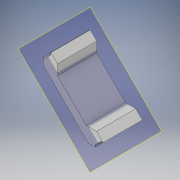
# Autodesk Inventor part: 20_Cube_Insert_Mirror_Holder_wLogo_v3
Saved by Autodesk Inventor 2019 (Build 230136000, 136)
## iProperties
Created: 2019-07-22
Part Number: 20_Cube_Insert_Mirror_Holder_wLogo_v3
Material: Generic
Document SubType Name: Modeling
Designer: diederichbenedict
Density: 1 g/cm^3
Appearance: Default
Mass: 13.6419 g
Surface Area: 50.8514 cm^2
Volume: 13.6419 cm^3
Author: diederichbenedict
Autodesk Inventor part; units mm, degrees
ref_plane "YZ Plane" through (0, 0, 0) normal (1, 0, 0) x (0, 1, 0)
ref_plane "XZ Plane" through (0, 0, 0) normal (0, 1, 0) x (-1, 0, 0)
ref_plane "XY Plane" through (0, 0, 0) normal (0, 0, 1) x (1, 0, 0)
sketch "Sketch1" plane through (0, 0, 0) normal (0, 0, 1) x (1, 0, 0)
  line L0 (-16.9, 21.4) -> (-16.9, 16.9) construction
  arc A0 (-22.9, 19.9) -> (-19.9, 22.9) centre (-19.9, 19.9) ccw construction
  line L1 (-16.9, 16.9) -> (16.9, 16.9) construction
  line L2 (16.9, 16.9) -> (16.9, -16.9) construction
  line L3 (16.9, -16.9) -> (-16.9, -16.9) construction
  line L4 (-16.9, -16.9) -> (-16.9, 16.9) construction
  arc A1 (22.9, -19.9) -> (19.9, -22.9) centre (19.9, -19.9) ccw construction
  line L5 (22.9, 19.9) -> (22.9, -19.9) construction
  arc A2 (19.9, 22.9) -> (22.9, 19.9) centre (19.9, 19.9) ccw construction
  line L6 (-19.9, 22.9) -> (19.9, 22.9) construction
  arc A3 (-22.9, 19.9) -> (-19.9, 22.9) centre (-19.9, 19.9) ccw construction
  line L7 (-22.9, -19.9) -> (-22.9, 19.9) construction
  arc A4 (-19.9, -22.9) -> (-22.9, -19.9) centre (-19.9, -19.9) ccw construction
  line L8 (19.9, -22.9) -> (-19.9, -22.9) construction
  line L9 (-21.4, 16.9) -> (-16.9, 16.9) construction
  line L10 (-16.9, -16.9) -> (-21.4, -16.9) construction
  line L11 (-16.9, -16.9) -> (-16.9, -21.4) construction
  line L12 (16.9, -21.4) -> (16.9, -16.9) construction
  line L13 (21.4, -16.9) -> (16.9, -16.9) construction
  line L14 (16.9, 16.9) -> (21.4, 16.9) construction
  line L15 (16.9, 16.9) -> (16.9, 21.4) construction
  line L16 (-16.8009, 21.2415) -> (21.2415, -16.8009)
  line L17 (21.2415, -16.8009) -> (16.8009, -21.2415)
  line L18 (16.8009, -21.2415) -> (-21.2415, 16.8009)
  line L19 (-21.2415, 16.8009) -> (-16.8009, 21.2415)
  line L20 (-16.8009, 21.2415) -> (16.8009, -21.2415) construction
  line L21 (21.2415, -16.8009) -> (-21.2415, 16.8009) construction
  line L22 (-16.8009, 21.2415) -> (36.9991, 21.2415) construction
  line L23 (-21.2415, 16.8009) -> (-22.9, 16.8009)
  line L24 (16.8009, -21.2415) -> (16.8009, -22.9)
  line L25 (16.8009, -22.9) -> (-22.9, 16.8009)
  line L26 (-16.8009, 21.2415) -> (-16.8009, 22.9)
  line L27 (21.2415, -16.8009) -> (22.9, -16.8009)
  line L28 (22.9, -16.8009) -> (-16.8009, 22.9)
  line L29 (-22.9, 16.8009) -> (-22.9, 11.5863)
  line L30 (16.8009, -22.9) -> (11.5863, -22.9)
  line L31 (-22.9, 11.5863) -> (11.5863, -22.9)
  point P0 (0, 0)
  dimension "d0" = 53.8
  dimension "d1" = 45
  dimension "d2" = 6.28
  dimension "d5" = 8
  constraints: 32 end point, 6 point on line, 4 parallel, 4 perpendicular, 2 midpoint, 1 equal length, 1 horizontal
  measures "d0" distance of L16.start L16.end
  measures "d1" angle of L16 L22
  measures "d2" distance of L16.end L17.end
  measures "d5" distance from line of L31 point (0, 0)
extrude "Extrusion1" add sketch "Sketch1" along normal blind 30
ref_plane "Work Plane1" through (16.9, -16.9, -8) normal (-0.7071068, -0.7071068, 0) x (0, 0, 1)
sketch "Sketch7" plane through (0, 0, 30) normal (0, 0, 1) x (1, 0, 0)
  line L0 (21.2415, -16.8009) -> (22.9, -16.8009) projected
  line L1 (22.9, -16.8009) -> (-16.8009, 22.9) projected
  line L2 (-16.8009, 22.9) -> (-16.8009, 21.2415) projected
  line L3 (-16.8009, 21.2415) -> (-21.2415, 16.8009) projected
  line L4 (-21.2415, 16.8009) -> (-22.9, 16.8009) projected
  line L5 (-22.9, 16.8009) -> (-22.9, 11.5863) projected
  line L6 (-22.9, 11.5863) -> (11.5863, -22.9) projected
  line L7 (11.5863, -22.9) -> (16.8009, -22.9) projected
  line L8 (16.8009, -22.9) -> (16.8009, -21.2415) projected
  line L9 (16.8009, -21.2415) -> (21.2415, -16.8009) projected
  line L10 (3.0496, 3.0496) -> (-5.6569, -5.6569)
  line L11 (-22.9, 11.5863) -> (11.5863, -22.9) projected
  line L12 (17.9785, -3.9418) -> (10.0409, -11.8794)
  line L13 (10.0409, -11.8794) -> (-11.8794, 10.0409)
  line L14 (-11.8794, 10.0409) -> (-3.9418, 17.9785)
  line L15 (-3.9418, 17.9785) -> (17.9785, -3.9418)
  line L16 (17.9785, -3.9418) -> (-11.8794, 10.0409) construction
  line L17 (10.0409, -11.8794) -> (-3.9418, 17.9785) construction
  line L18 (-11.8794, 10.0409) -> (-11.8794, 17.9785)
  line L19 (22.9, -16.8009) -> (-16.8009, 22.9) projected
  line L20 (10.0409, -11.8794) -> (17.9785, -11.8794)
  point P0 (0, 0)
  dimension "d28" = 31
  dimension "d29" = 1.3
  constraints: 18 end point, 4 midpoint, 2 parallel, 2 perpendicular, 2 point on line, 1 vertical
  measures "d28" distance of L12.end L13.end
  measures "d29" distance from line of L13 point (0, 0)
extrude "Extrusion7" cut sketch "Sketch7" against normal through all contours L20 L12 L1 | L12 L13 L10 L1 | L1 L14 L15 L12 | L10 L13 L14 L1 | L14 L18 L1
sketch "Sketch10" plane through (11.5863, -22.9, 30) normal (-0.7071068, -0.7071068, 0) x (-0.7071068, 0.7071068, 0)
  line L0 (1.6838, 16.5215) -> (7.0744, 16.5215) construction
  line L1 (7.0744, 16.5215) -> (7.0744, 10.5304) construction
  line L2 (7.0744, 10.5304) -> (1.6838, 10.5304) construction
  line L3 (1.6838, 10.5304) -> (1.6838, 6.839) construction
  line L4 (1.6838, 6.839) -> (6.7206, 6.839) construction
  line L5 (6.7206, 6.839) -> (6.7206, 1.2092) construction
  line L6 (6.7206, 1.2092) -> (1.6838, 1.2092) construction
  line L7 (1.6838, 1.2092) -> (1.6838, -3.423) construction
  line L8 (1.6838, -3.423) -> (34.6838, -3.423) construction
  line L9 (34.6838, 30.377) -> (1.6838, 30.377) construction
  line L10 (1.6838, 30.377) -> (1.6838, 26.2152) construction
  line L11 (1.6838, 26.2152) -> (7.1181, 26.2152) construction
  line L12 (7.1181, 26.2152) -> (7.1181, 20.0634) construction
  line L13 (7.1181, 20.0634) -> (1.6838, 20.0634) construction
  line L14 (1.6838, 20.0634) -> (1.6838, 16.5215) construction
  line L15 (7.0744, 13.526) -> (34.6838, 13.477) construction
  line L16 (1.6838, 30.377) -> (36.6838, 30.377) construction
  line L17 (36.6838, -3.423) -> (1.6838, -3.423) construction
  line L18 (15.7252, 20) -> (15.7252, 10)
  line L19 (15.7252, 10) -> (24.3855, 5)
  line L20 (15.7252, 20) -> (17.2252, 19.134)
  line L21 (17.2252, 19.134) -> (17.2252, 10.866)
  line L22 (17.2252, 10.866) -> (22.8855, 7.5981)
  line L23 (22.8855, 7.5981) -> (22.8855, 15.866)
  line L24 (22.8855, 15.866) -> (24.3855, 15)
  line L25 (24.3855, 15) -> (24.3855, 5)
  line L26 (34.6838, 30.377) -> (34.6838, -3.423)
  line L27 (24.3855, 31.8785) -> (24.3855, -1.9215) construction
  line L28 (1.6838, -3.423) -> (34.6838, -3.423) construction
  line L29 (34.6838, 30.377) -> (34.6838, 30.377) construction
  line L30 (34.6838, 30.377) -> (34.6838, -3.423) construction
  line L31 (34.6838, -3.423) -> (34.6838, -3.423) construction
  line L32 (34.6838, -3.423) -> (34.6838, 30.377) construction
  line L33 (48.771, 30) -> (0, 30) construction
  line L34 (0, 30) -> (0, 0) construction
  line L35 (48.771, 0) -> (0, 0) construction
  line L36 (48.771, 30) -> (48.771, 0) construction
  line L37 (24.3855, 30) -> (24.3855, 0) construction
  line L38 (48.771, 0) -> (0, 0) construction
  line L39 (48.771, 30) -> (48.771, 0) construction
  line L40 (48.771, 15) -> (0, 15) construction
  line L41 (0, 30) -> (0, 0) construction
  point P0 (24.3855, 15)
  dimension "d40" = 1.5
  dimension "d41" = 1.5
  dimension "d42" = 1.5
  dimension "d43" = 10
  dimension "d44" = 10
  constraints: 70 end point, 6 midpoint, 4 parallel, 3 collinear, 1 perpendicular, 1 vertical
  measures "d40" distance between parallel lines of L21 L18
  measures "d41" distance between parallel lines of L25 L23
  measures "d42" distance between parallel lines of L19 L22
  measures "d43" distance of L18.start L18.end
  measures "d44" distance of L18.end L19.end
emboss "Emboss1" sketch "Sketch10" operation cut depth 1 direction (0.7071068, 0.7071068, 0)
sketch "Sketch11" plane through (11.5863, -22.9, 30) normal (-0.7071068, -0.7071068, 0) x (-0.7071068, 0.7071068, 0)
  line L0 (17.2252, 10.866) -> (22.8855, 7.5981) construction
  line L1 (22.8855, 7.5981) -> (22.8855, 15.866) construction
  line L2 (22.8855, 15.866) -> (24.3855, 15) construction
  line L3 (24.3855, 15) -> (24.3855, 5) construction
  line L4 (24.3855, 5) -> (15.7252, 10) construction
  line L5 (15.7252, 10) -> (15.7252, 20) construction
  line L6 (15.7252, 20) -> (17.2252, 19.134) construction
  line L7 (17.2252, 19.134) -> (17.2252, 10.866) construction
  line L8 (48.771, 30) -> (0, 30) construction
  line L9 (0, 30) -> (0, 0) construction
  line L10 (48.771, 0) -> (0, 0) construction
  line L11 (48.771, 30) -> (48.771, 0) construction
  line L12 (15.7252, 20) -> (17.2252, 19.134) construction
  line L13 (17.2252, 19.134) -> (17.2252, 10.866) construction
  line L14 (17.2252, 10.866) -> (22.8855, 7.5981) construction
  line L15 (22.8855, 7.5981) -> (22.8855, 15.866) construction
  line L16 (22.8855, 15.866) -> (24.3855, 15) construction
  line L17 (24.3855, 15) -> (24.3855, 5) construction
  line L18 (24.3855, 5) -> (15.7252, 10) construction
  line L19 (15.7252, 10) -> (15.7252, 20) construction
  line L20 (15.5651, 18.4016) -> (15.5, -16.9) construction
  line L21 (15.5651, 18.4016) -> (-17.5, 16.9) construction
  line L22 (-17.5, 16.9) -> (-17.5, 12.7382) construction
  line L23 (-17.5, 12.7382) -> (-12.0658, 12.7382) construction
  line L24 (-12.0658, 12.7382) -> (-12.0658, 6.5864) construction
  line L25 (-12.0658, 6.5864) -> (-17.5, 6.5864) construction
  line L26 (-17.5, 6.5864) -> (-17.5, 3.0446) construction
  line L27 (-17.5, 3.0446) -> (-12.1095, 3.0446) construction
  line L28 (-12.1095, 3.0446) -> (-12.1095, -2.9465) construction
  line L29 (-12.1095, -2.9465) -> (-17.5, -2.9465) construction
  line L30 (-17.5, -2.9465) -> (-17.5, -6.638) construction
  line L31 (-17.5, -6.638) -> (-12.4632, -6.638) construction
  line L32 (-12.4632, -6.638) -> (-12.4632, -12.2678) construction
  line L33 (-12.4632, -12.2678) -> (-17.5, -12.2678) construction
  line L34 (-17.5, -12.2678) -> (-17.5, -16.9) construction
  line L35 (-17.5, -16.9) -> (15.5, -16.9) construction
  line L36 (-12.1095, 0.049) -> (15.5326, 0.7508) construction
  line L37 (15.5, -16.9) -> (15.5651, 18.4016) construction
  line L38 (1.91, 17.7815) -> (1.91, -16.9) construction
  line L39 (15.5, -16.9) -> (-17.5, -16.9) construction
  line L40 (22.8855, 7.5981) -> (22.8855, 15.866) construction
  line L41 (17.2252, 19.134) -> (17.2252, 10.866)
  line L42 (17.2252, 10.866) -> (22.8855, 7.5981)
  line L43 (17.2252, 19.134) -> (17.2252, 10.866)
  line L44 (17.2252, 10.866) -> (22.8855, 7.5981)
  line L45 (22.8855, 7.5981) -> (22.8855, 9.3301)
  line L46 (22.8855, 7.5981) -> (22.8855, 15.866)
  line L47 (22.8855, 9.3301) -> (18.7252, 11.7321)
  line L48 (18.7252, 11.7321) -> (18.7252, 18.2679)
  line L49 (18.7252, 18.2679) -> (22.8855, 20.6699)
  line L50 (17.2252, 19.134) -> (22.8855, 22.4019)
  line L51 (22.8855, 22.4019) -> (22.8855, 20.6699)
  point P0 (24.3855, 30)
  point P1 (20.9754, 14.9785)
  dimension "d47" = 120
  dimension "d48" = 1.5
  dimension "d49" = 1.5
  dimension "d50" = 1.5
  constraints: 80 end point, 5 parallel, 3 point on line, 2 collinear, 2 midpoint
  measures "d47" angle of L50 L12
  measures "d48" distance between parallel lines of L13 L48
  measures "d49" distance between parallel lines of L50 L49
  measures "d50" distance between parallel lines of L14 L47
emboss "Emboss2" sketch "Sketch11" operation cut depth 1.5 direction (0.7071068, 0.7071068, 0)
sketch "Sketch12" plane through (11.5863, -22.9, 30) normal (-0.7071068, -0.7071068, 0) x (-0.7071068, 0.7071068, 0)
  line L0 (18.7252, 11.7321) -> (22.8855, 9.3301) construction
  line L1 (22.8855, 9.3301) -> (22.8855, 15.866) construction
  line L2 (22.8855, 15.866) -> (24.3855, 15) construction
  line L3 (24.3855, 15) -> (24.3855, 5) construction
  line L4 (24.3855, 5) -> (15.7252, 10) construction
  line L5 (15.7252, 10) -> (15.7252, 20) construction
  line L6 (15.7252, 20) -> (17.2252, 19.134) construction
  line L7 (17.2252, 19.134) -> (22.8855, 22.4019) construction
  line L8 (22.8855, 22.4019) -> (22.8855, 20.6699) construction
  line L9 (22.8855, 20.6699) -> (18.7252, 18.2679) construction
  line L10 (18.7252, 18.2679) -> (18.7252, 11.7321) construction
  line L11 (48.771, 30) -> (0, 30) construction
  line L12 (0, 30) -> (0, 0) construction
  line L13 (48.771, 0) -> (0, 0) construction
  line L14 (48.771, 30) -> (48.771, 0) construction
  line L15 (18.7252, 11.7321) -> (22.8855, 9.3301) construction
  line L16 (22.8855, 9.3301) -> (22.8855, 15.866) construction
  line L17 (22.8855, 15.866) -> (24.3855, 15) construction
  line L18 (24.3855, 15) -> (24.3855, 5) construction
  line L19 (24.3855, 5) -> (15.7252, 10) construction
  line L20 (15.7252, 10) -> (15.7252, 20) construction
  line L21 (15.7252, 20) -> (17.2252, 19.134) construction
  line L22 (17.2252, 19.134) -> (22.8855, 22.4019) construction
  line L23 (22.8855, 22.4019) -> (22.8855, 20.6699) construction
  line L24 (22.8855, 20.6699) -> (18.7252, 18.2679) construction
  line L25 (18.7252, 18.2679) -> (18.7252, 11.7321) construction
  line L26 (15.5651, 18.4016) -> (15.5, -16.9) construction
  line L27 (15.5651, 18.4016) -> (-17.5, 16.9) construction
  line L28 (-17.5, 16.9) -> (-17.5, 12.7382) construction
  line L29 (-17.5, 12.7382) -> (-12.0658, 12.7382) construction
  line L30 (-12.0658, 12.7382) -> (-12.0658, 6.5864) construction
  line L31 (-12.0658, 6.5864) -> (-17.5, 6.5864) construction
  line L32 (-17.5, 6.5864) -> (-17.5, 3.0446) construction
  line L33 (-17.5, 3.0446) -> (-12.1095, 3.0446) construction
  line L34 (-12.1095, 3.0446) -> (-12.1095, -2.9465) construction
  line L35 (-12.1095, -2.9465) -> (-17.5, -2.9465) construction
  line L36 (-17.5, -2.9465) -> (-17.5, -6.638) construction
  line L37 (-17.5, -6.638) -> (-12.4632, -6.638) construction
  line L38 (-12.4632, -6.638) -> (-12.4632, -12.2678) construction
  line L39 (-12.4632, -12.2678) -> (-17.5, -12.2678) construction
  line L40 (-17.5, -12.2678) -> (-17.5, -16.9) construction
  line L41 (-17.5, -16.9) -> (15.5, -16.9) construction
  line L42 (17.2252, 19.134) -> (22.8855, 22.4019)
  line L43 (15.7252, 20) -> (17.2252, 19.134)
  line L44 (17.2252, 19.134) -> (22.8855, 22.4019)
  line L45 (22.8855, 22.4019) -> (22.8855, 20.6699)
  line L46 (22.8855, 22.4019) -> (22.8855, 20.6699)
  line L47 (22.8855, 31.8785) -> (22.8855, -1.9215) construction
  line L48 (22.8855, 9.3301) -> (22.8855, 15.866) construction
  line L49 (15.7252, 20) -> (22.8855, 24.134)
  line L50 (22.8855, 24.134) -> (31.5457, 19.134)
  line L51 (31.5457, 19.134) -> (31.5457, 17.4019)
  line L52 (31.5457, 17.4019) -> (25.8855, 14.134)
  line L53 (25.8855, 14.134) -> (25.8855, 9.3301)
  line L54 (25.8855, 9.3301) -> (30.0457, 11.7321)
  line L55 (31.5457, 9.134) -> (31.5457, 9.134)
  line L56 (24.3855, 5) -> (15.7252, 10)
  line L57 (31.5457, 9.134) -> (24.3855, 5)
  line L58 (22.8855, 15.866) -> (24.3855, 15)
  line L59 (24.3855, 5) -> (24.3855, 15)
  line L60 (24.3855, 15) -> (22.8855, 15.866)
  line L61 (22.8855, 20.6699) -> (18.7252, 18.2679)
  line L62 (22.8855, 20.6699) -> (22.8855, 22.4019)
  line L63 (24.3855, 15) -> (24.3855, 5)
  line L64 (22.8855, 15.866) -> (27.0457, 18.2679)
  line L65 (27.0457, 18.2679) -> (22.8855, 20.6699)
  line L66 (15.7252, 10) -> (24.3855, 5) construction
  line L67 (18.7252, 11.7321) -> (22.8855, 9.3301) construction
  line L68 (18.7252, 11.7321) -> (24.3855, 8.4641) construction
  line L69 (24.3855, 8.4641) -> (34.3988, 14.2453) construction
  line L70 (24.3855, 15) -> (31.5457, 19.134) construction
  line L71 (24.3855, 5) -> (39.2099, 13.5589) construction
  line L72 (27.0457, 18.2679) -> (31.2025, 17.6001) construction
  line L73 (22.8855, 22.4019) -> (22.8855, 20.6699) construction
  line L74 (31.2025, 17.6001) -> (22.8855, 22.4019) construction
  line L75 (31.5457, 9.134) -> (31.5457, 10.866)
  line L76 (31.5457, 10.866) -> (30.0457, 11.7321)
  line L77 (18.7252, 11.7321) -> (22.8855, 9.3301) construction
  line L78 (18.7252, 18.2679) -> (18.7252, 11.7321) construction
  line L79 (22.8855, 20.6699) -> (18.7252, 18.2679) construction
  line L80 (22.8855, 22.4019) -> (22.8855, 20.6699) construction
  line L81 (17.2252, 19.134) -> (22.8855, 22.4019) construction
  line L82 (17.2252, 10.866) -> (17.2252, 19.134) construction
  line L83 (22.8855, 7.5981) -> (17.2252, 10.866) construction
  line L84 (22.8855, 9.3301) -> (22.8855, 7.5981) construction
  line L85 (22.8855, 7.5981) -> (24.3855, 6.7321) construction
  line L86 (24.3855, 6.7321) -> (34.2349, 12.4186) construction
  point P0 (24.3855, 30)
  point P1 (20.9754, 14.9785)
  dimension "d54" = 60
  dimension "d55" = 1.5
  dimension "d56" = 120
  dimension "d57" = 120
  dimension "d58" = 1.5
  dimension "d59" = 120
  constraints: 144 end point, 11 parallel, 6 collinear, 6 point on line, 2 vertical, 2 other
  measures "d54" angle of L21 L49
  measures "d55" distance between parallel lines of L53 L18
  measures "d56" angle of L47 L50
  measures "d57" angle of L18 L69
  measures "d58" distance between parallel lines of L70 L52
  measures "d59" angle of L75 L76
extrude "Extrusion9" cut sketch "Sketch12" against normal blind 2
sketch "Sketch13" plane through (0, 0, 30) normal (0, 0, 1) x (1, 0, 0)
  line L0 (-11.8794, 10.0409) -> (-11.8794, 17.9785) construction
  line L1 (-11.8794, 17.9785) -> (-16.8009, 22.9) construction
  line L2 (-16.8009, 22.9) -> (-16.8009, 21.2415) projected
  line L3 (-16.8009, 21.2415) -> (-21.2415, 16.8009) projected
  line L4 (-21.2415, 16.8009) -> (-22.9, 16.8009) projected
  line L5 (-22.9, 16.8009) -> (-22.9, 11.5863) construction
  line L6 (-22.9, 11.5863) -> (11.5863, -22.9) construction
  line L7 (11.5863, -22.9) -> (16.8009, -22.9) construction
  line L8 (16.8009, -22.9) -> (16.8009, -21.2415) projected
  line L9 (16.8009, -21.2415) -> (21.2415, -16.8009) projected
  line L10 (21.2415, -16.8009) -> (22.9, -16.8009) projected
  line L11 (22.9, -16.8009) -> (17.9785, -11.8794) construction
  line L12 (17.9785, -11.8794) -> (10.0409, -11.8794) construction
  line L13 (10.0409, -11.8794) -> (-11.8794, 10.0409) construction
  line L14 (-11.7794, 10.0823) -> (-11.7794, 18.02) construction
  line L15 (-11.7794, 18.02) -> (-16.9009, 23.1414) construction
  line L16 (-16.9009, 23.1414) -> (-16.9009, 21.2829)
  line L17 (-16.9009, 21.2829) -> (-21.2829, 16.9009)
  line L18 (-21.2829, 16.9009) -> (-23, 16.9009)
  line L19 (-23, 16.9009) -> (-23, 11.5449) construction
  line L20 (-23, 11.5449) -> (11.5449, -23) construction
  line L21 (11.5449, -23) -> (16.9009, -23) construction
  line L22 (16.9009, -23) -> (16.9009, -21.2829)
  line L23 (16.9009, -21.2829) -> (21.2829, -16.9009)
  line L24 (21.2829, -16.9009) -> (23.1414, -16.9009)
  line L25 (23.1414, -16.9009) -> (18.02, -11.7794) construction
  line L26 (18.02, -11.7794) -> (10.0823, -11.7794) construction
  line L27 (10.0823, -11.7794) -> (-11.7794, 10.0823) construction
  line L28 (16.8009, -22.9) -> (16.9009, -22.9)
  line L29 (22.9, -16.8009) -> (23, -16.9009)
  line L30 (-21.2415, 16.8009) -> (-22.9, 16.8009) projected
  line L31 (-22.9, 16.8009) -> (-22.9, 16.9009)
  line L32 (-16.8009, 22.9) -> (-16.9009, 23)
  point P0 (0, 0)
  dimension "d65" = 0.1
  constraints: 36 end point, 5 point on line, 2 perpendicular, 13 other
  measures "d65" distance between parallel lines of L13 L27
extrude "IM_offset" add sketch "Sketch13" against normal up to surface (30 mm away)
equation "\"d3\" = MirrorThickness1"
equation "\"d41\" = d40"
equation "\"d42\" = d40"
equation "\"d44\" = d43"
equation "\"d48\" = d51"
equation "\"d49\" = d51"
equation "\"d50\" = d51"
equation "\"d55\" = d60"
equation "\"d58\" = d60"
equation "\"MirrorThickness1\" = 30"
equation "\"d51\" = 1.5"
equation "\"d60\" = 1.5"
body "Solid1"
